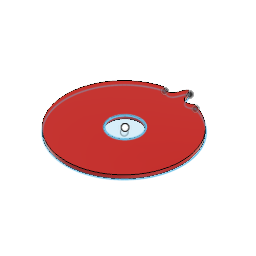
Wheel with Spike (Autodesk Fusion 360 design; units mm, degrees)
Autodesk Fusion 360 part; units mm, degrees
sketch "sketch 404" plane through (0, 0, 0) normal (0, 0, 1) x (1, 0, 0)
  spline S0 degree 3 poles (48.9514, 101.0683) (48.479, 100.6398) (48.0603, 100.2994) (47.6389, 99.6736) (47.1764, 98.987) (46.7279, 97.934) (46.2918, 96.7404) (45.7147, 95.1607) (45.1444, 93.4403) (44.2162, 92.2772) (43.6032, 91.5091) (42.8015, 90.9859) (41.9732, 90.7882) (40.8489, 90.5198) (39.7714, 90.7639) (38.8442, 91.1249) (37.6862, 91.5756) (36.7344, 92.2267) (36.0375, 92.8278) (36.0026, 92.8579) (35.9683, 92.888) (35.9346, 92.918) knots 0.083994 0.083994 0.083994 0.083994 0.199846 0.199846 0.199846 0.326977 0.326977 0.326977 0.495233 0.495233 0.495233 0.606356 0.606356 0.606356 0.757203 0.757203 0.757203 0.945577 0.945577 0.945577 0.955014 0.955014 0.955014 0.955014
  arc A0 (35.9346, 92.918) -> (61.9683, 92.918) centre (48.9514, 45.6786) ccw
  spline S1 degree 3 poles (48.9514, 101.0683) (49.4238, 100.6398) (49.8426, 100.2994) (50.264, 99.6736) (50.7264, 98.987) (51.175, 97.934) (51.611, 96.7404) (52.1881, 95.1607) (52.7585, 93.4403) (53.6866, 92.2772) (54.2996, 91.5091) (55.1014, 90.9859) (55.9296, 90.7882) (57.054, 90.5198) (58.1314, 90.7639) (59.0587, 91.1249) (60.2167, 91.5756) (61.1684, 92.2267) (61.8653, 92.8278) (61.9003, 92.8579) (61.9346, 92.888) (61.9683, 92.918) knots 0.083994 0.083994 0.083994 0.083994 0.199846 0.199846 0.199846 0.326977 0.326977 0.326977 0.495233 0.495233 0.495233 0.606356 0.606356 0.606356 0.757203 0.757203 0.757203 0.945577 0.945577 0.945577 0.955014 0.955014 0.955014 0.955014
extrude "Extrude1" add sketch "sketch 404" along normal blind 3
hole "Hole1" at (48.782, 46.5698, 3) direction (0, 0, -1) diameter 25 depth 25 tip angle 118
sketch "sketch 431" plane through (0, 0, 3) normal (0, 0, 1) x (-1, 0, 0)
  circle A0 centre (-48.782, -46.5698) radius 12.5
  circle A1 centre (-48.782, -46.5698) radius 12.5
extrude "Extrude2" add sketch "sketch 431" against normal blind 36
sketch "sketch 446" plane through (0, 0, 3) normal (0, 0, 1) x (-1, 0, 0)
  circle A0 centre (-48.782, -46.5698) radius 12.5
  circle A1 centre (-48.782, -46.5698) radius 12.5
extrude "Extrude3" cut sketch "sketch 446" against normal blind 51
